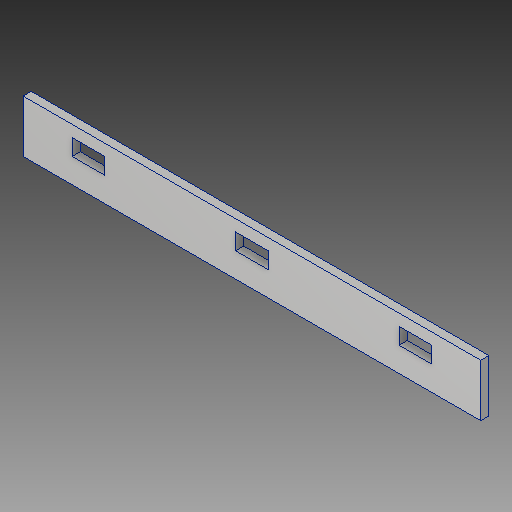
# Autodesk Inventor part: latchplate
Saved by Autodesk Inventor 2018.1 (Build 221171000, 171)
## iProperties
Created: 2017-08-11
Part Number: latchplate
Material: Aluminum 6061
Document SubType Name: Modeling
Designer: Kai
Density: 2.7 g/cm^3
Appearance: Aluminum - Flat
Author: Kai
Autodesk Inventor part; units mm, degrees
ref_plane "YZ Plane" through (0, 0, 0) normal (1, 0, 0) x (0, 1, 0)
ref_plane "XZ Plane" through (0, 0, 0) normal (0, 1, 0) x (-1, 0, 0)
ref_plane "XY Plane" through (0, 0, 0) normal (0, 0, 1) x (1, 0, 0)
sketch "Sketch1" plane through (0, 0, 0) normal (0, 0, 1) x (1, 0, 0)
  line L0 (0, 0) -> (355.6, 0)
  line L1 (355.6, 0) -> (355.6, 40.64)
  line L2 (355.6, 40.64) -> (0, 40.64)
  line L3 (0, 40.64) -> (0, 0)
  line L4 (0, 31.75) -> (355.6, 31.75) construction
  line L5 (38.1, 31.75) -> (63.5, 31.75)
  line L6 (63.5, 31.75) -> (63.5, 19.05)
  line L7 (63.5, 19.05) -> (38.1, 19.05)
  line L8 (38.1, 19.05) -> (38.1, 31.75)
  line L9 (317.5, 31.75) -> (292.1, 31.75)
  line L10 (292.1, 31.75) -> (292.1, 19.05)
  line L11 (292.1, 19.05) -> (317.5, 19.05)
  line L12 (317.5, 19.05) -> (317.5, 31.75)
  line L13 (165.1, 31.75) -> (190.5, 31.75)
  line L14 (190.5, 31.75) -> (190.5, 19.05)
  line L15 (190.5, 19.05) -> (165.1, 19.05)
  line L16 (165.1, 19.05) -> (165.1, 31.75)
  dimension "d0" = 355.6
  dimension "d1" = 40.64
  dimension "d2" = 8.89
  dimension "d3" = 25.4
  dimension "d4" = 12.7
  dimension "d5" = 38.1
  dimension "d6" = 25.4
  dimension "d7" = 12.7
  dimension "d8" = 25.4
  dimension "d9" = 12.7
  dimension "d10" = 38.1
  dimension "d11" = 165.1
  constraints: 34 end point, 8 parallel, 5 perpendicular, 5 point on line, 4 horizontal
  measures "d0" distance of L2.end L1.end
  measures "d1" distance of L1.end L0.end
  measures "d2" distance between parallel lines of L2 L4
  measures "d3" distance of L6.end L7.end
  measures "d4" distance of L5.end L6.end
  measures "d5" distance between parallel lines of L3 L8
  measures "d6" distance of L11.end L10.end
  measures "d7" distance of L10.end L9.end
  measures "d8" distance of L14.end L15.end
  measures "d9" distance of L13.end L14.end
  measures "d10" distance from line of L11.end L1
  measures "d11" distance between parallel lines of L1 L14
extrude "Extrusion1" add sketch "Sketch1" along normal blind 6.35
body "Solid1"
